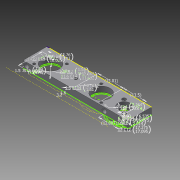
# Autodesk Inventor part: mount
Saved by Autodesk Inventor 2014 (Build 180170000, 170)
## iProperties
Created: 2013-09-13
Part Number: mount
Material: Generic
Document SubType Name: Modeling
Designer: Brandon
Density: 1 g/cm^3
Appearance: Default
Author: Brandon
Autodesk Inventor part; units mm, degrees
ref_plane "YZ Plane" through (0, 0, 0) normal (1, 0, 0) x (0, 1, 0)
ref_plane "XZ Plane" through (0, 0, 0) normal (0, 1, 0) x (-1, 0, 0)
ref_plane "XY Plane" through (0, 0, 0) normal (0, 0, 1) x (1, 0, 0)
sketch "Sketch1" plane through (0, 0, 0) normal (0, 0, 1) x (1, 0, 0)
  circle A0 centre (0, 0) radius 0.88
  circle A1 centre (-13, 0) radius 6.031
  line L0 (0, 7.8471) -> (0, -6.1529)
  line L1 (-22.031, -6.1529) -> (35.1375, -6.1529)
  line L2 (-22.031, 7.8471) -> (-22.031, -6.1529)
  circle A2 centre (-13, 0) radius 5.1925
  line L3 (-13, 0) -> (-9.1435, 0) construction
  line L4 (-13, 0) -> (-8.3268, 0) construction
  circle A3 centre (-8.1698, 4.8302) radius 0.775
  circle A4 centre (-17.8302, -4.8302) radius 0.75
  circle A5 centre (13, 0) radius 6.031
  circle A6 centre (13, 0) radius 5.1925
  line L5 (13, 0) -> (9.1435, 0) construction
  line L6 (13, 0) -> (8.3268, 0) construction
  circle A7 centre (8.1698, 4.8302) radius 0.775
  circle A8 centre (17.8302, -4.8302) radius 0.75
  line L7 (13, 0) -> (-13, 0)
  circle A9 centre (26.5, 0) radius 4.5 construction
  circle A10 centre (26.5, 0) radius 8.6375
  line L8 (26.5, 0) -> (30.5894, 0) construction
  circle A11 centre (22.8938, 3.6062) radius 1.132
  circle A12 centre (30.1062, -3.6062) radius 1.132
  line L9 (0, -6.1529) -> (-0.0044, -7.7529) construction
  line L10 (-0.0044, -7.7529) -> (-19.5609, -7.6995) construction
  line L11 (-0.0044, -7.7529) -> (19.5522, -7.8064) construction
  circle A13 centre (13, 0) radius 9 construction
  circle A14 centre (26.5, 0) radius 2.5 construction
  circle A15 centre (26.5, 0) radius 3.2675
  line L12 (13, 0) -> (26.5, 0)
  line L13 (30.1062, -3.6062) -> (22.8938, 3.6062) construction
  line L14 (33.2882, -0.4243) -> (26.0757, 6.7882)
  line L15 (19.7118, 0.4243) -> (26.9243, -6.7882)
  arc A16 (26.9243, -6.7882) -> (33.2882, -0.4243) centre (30.1062, -3.6062) ccw
  arc A17 (26.0757, 6.7882) -> (19.7118, 0.4243) centre (22.8938, 3.6062) ccw
  circle A18 centre (26.5, 0) radius 7.7
  circle A19 centre (26.5, 0) radius 3.5
  line L16 (-22.031, 7.8471) -> (35.1375, 7.8471)
  line L17 (35.1375, 7.8471) -> (35.1375, -6.1529)
  line L18 (20.438, -6.1529) -> (32.562, -6.1529) construction
  line L19 (-0.0044, -7.7529) -> (-0.0007, -10.9529) construction
  line L20 (-0.0007, -10.9529) -> (30.0115, -10.9189) construction
  line L21 (-0.0007, -10.9529) -> (-30.0007, -10.9869) construction
  line L22 (-0.0007, -10.9529) -> (29.9993, -10.9529) construction
  circle A20 centre (0, 0) radius 4 construction
  line L23 (-13, 0) -> (-8.7354, 4.2646) construction
  line L24 (-13, 0) -> (-17.2646, -4.2646) construction
  line L25 (-8.7354, 4.2646) -> (-8.1698, 4.8302) construction
  line L26 (-17.2646, -4.2646) -> (-17.8302, -4.8302) construction
  line L27 (-17.2646, -4.2646) -> (-16.4646, -4.2646) construction
  circle A21 centre (13, 0) radius 12 construction
  circle A22 centre (-13, 0) radius 12 construction
  line L28 (1, 0) -> (-1, 0) construction
  line L29 (-19.031, 0) -> (-22.031, 0) construction
  dimension "d105" = 24
  dimension "d106" = 24
  dimension "d0" = 1.5
  dimension "d3" = 11.6
  dimension "d8" = 10
  dimension "d13" = 1.5
  dimension "d14" = 1.5
  dimension "d26" = 17
  dimension "d31" = 2
  dimension "d32" = 2
  dimension "d38" = 5
  dimension "d40" = 6.15
  dimension "d42" = 13
  dimension "d52" = 13.5
  dimension "d53" = 9
  dimension "d54" = 7
  dimension "d60" = 12.124
  dimension "d81" = 1.6
  dimension "d86" = 3.2
  dimension "d87" = 45
  dimension "d88" = 10.2
  dimension "d89" = 8
  dimension "d90" = 0.8
  dimension "d91" = 0.8
  dimension "d92" = 135
  dimension "d98" = 14
  dimension "d103" = 18
  dimension "d104" = 9
  dimension "d107" = 2
  dimension "d108" = 3
  constraints: 62 end point, 21 centre point, 15 coincident, 9 point on circle, 8 horizontal, 7 collinear, 7 point on line, 7 tangent, 6 symmetric about line, 4 perpendicular, 2 equal length, 2 horizontal alignment, 2 midpoint, 1 parallel, 8 other
  measures "d14" diameter of A4
  measures "d38" diameter of A14
  measures "d42" distance of point (0, 0) A5.centre
  measures "d52" distance of L12.start L8.start
  measures "d53" diameter of A17
  measures "d54" diameter of A19
  measures "d60" distance of L18.start L18.end
  measures "d81" distance of L9.end L0.end
  measures "d86" distance of L9.end L19.end
  measures "d87" angle of L8 L13
  measures "d88" distance of L13.start L13.end
  measures "d89" diameter of A20
  measures "d90" distance of L23.end L25.end
  measures "d91" distance of L24.end L26.end
  measures "d92" angle of L26 L27
  measures "d98" distance of L2.start L1.start
  measures "d103" diameter of A13
  measures "d104" diameter of A9
  measures "d107" distance of L28.start L28.end
  measures "d108" distance of L29.start L29.end
extrude "Extrusion5" add sketch "Sketch1" along normal blind 4 contours L7 L0 A0 | L7 A5 A10 L1 L0 A0 | A0 L0 L16 A17 A10 A5 L7 | A0 L0 L7 | L0 L7 A0 | A0 L0 L1 L2 L16 | A0 L7 L0 | L7 A6 A10 A5 | A5 A10 A6 L7 | A10 A17 A5 | A5 A18 L12 A6 A10 | A10 A6 L12 A18 A5 | A5 A18 L1 A10 | L16 A10 A17 | A17 A18 A5 | A17 A10 L16 A18 | A18 L12 A5 | A5 L12 L15 L1 A18 | A18 A17 L15 L12 A5 | A5 L12 A18 | A18 A17 L14 A16 L1 L15 | L16 L17 A10 | A10 A16 A18 A17 L16 | A10 A16 L1 | L1 A18 A16 A10 | A16 A10 L17 L1 | A18 A16 L14 A17 | A1 picked at (20.7047, 6.7683) picked at (33.2521, -5.8435) picked at (32.0585, -5.7172)
extrude "Extrusion6" add sketch "Sketch1" along normal blind 0.6 contours A19
extrude "Extrusion7" add sketch "Sketch1" against normal blind 1 contours A18 L12 A5 | A5 L12 L15 L1 A18 | L1 L15 A16 A18 | A18 A17 L15 L12 A5 | A5 L12 A18 | A18 A17 L14 A16 L1 L15 | L1 A18 A16 L15 | A18 A16 L14 A17 | A19
extrude "Extrusion8" add sketch "Sketch1" against normal blind 2 contours L16 A10 A17 | A17 A10 L16 | A17 A10 L16 A18 | A17 L16 A10 | A16 A18 L1 A10 | A10 L1 A16 | A18 A17 L14 A16 L1 L15 | L1 A18 A16 L15 | A10 A16 L1 | L1 A18 A16 A10 | A19 picked at (20.7047, 6.7683) picked at (22.1116, 7.9072) picked at (23.7903, 7.8802) picked at (31.146, -6.8855) picked at (29.1888, -6.3623) picked at (32.0585, -5.7172)
extrude "Extrusion9" cut sketch "Sketch1" against normal up to surface (1 mm away) from surface at -1 contours A10 A17 A5 | A5 A18 L12 A6 A10 | A10 A6 L12 A18 A5 | A5 A18 L1 A10 | A17 A18 A5 | A17 A10 L16 A18 | A6 L12 A10 | A18 L12 A5 | A5 L12 L15 L1 A18 | A10 L12 A6 | A17 L16 A10 | A10 L16 A17 | A18 A17 L15 L12 A5 | A5 L12 A18 | A18 A17 L14 A16 L1 L15 | A10 A16 A18 A17 L16 | L1 A18 A16 A10 | A18 A16 L14 A17 | A19 picked at (23.7903, 7.8802) picked at (27.6663, 8.0331) picked at (32.0585, -5.7172)
extrude "Extrusion10" cut sketch "Sketch1" against normal blind 2 contours L7 L0 A0 | L7 A5 A10 L1 L0 A0 | A0 L0 L16 A17 A10 A5 L7 | A0 L0 L7 | A10 A17 A5 | A5 A18 L1 A10 | L16 A10 A17 | A17 A18 A5 | A17 A10 L16 A18 | A5 L12 L15 L1 A18 | A18 A17 L15 L12 A5 | A18 A17 L14 A16 L1 L15 | L16 L17 A10 | A10 A16 A18 A17 L16 | A10 A16 L1 | L1 A18 A16 A10 | A16 A10 L17 L1 | A18 A16 L14 A17 keep common part picked at (0.4122, 0.4122) picked at (0.4122, -0.4122) picked at (20.7047, 6.7683) picked at (33.2521, -5.8435) picked at (32.0585, -5.7172)
extrude "Extrusion11" add sketch "Sketch1" along normal blind 4 contours L7 L0 A0 | L7 A5 A10 L1 L0 A0 | A0 L0 L16 A17 A10 A5 L7 | A0 L0 L7 | L0 L7 A0 | A0 L0 L1 L2 L16 | A0 L7 L0 | L7 A6 A10 A5 | A5 A10 A6 L7 | A10 A17 A5 | A5 A18 L12 A6 A10 | A10 A6 L12 A18 A5 | A5 A18 L1 A10 | L16 A10 A17 | A17 A18 A5 | A17 A10 L16 A18 | A18 L12 A5 | A5 L12 L15 L1 A18 | A18 A17 L15 L12 A5 | A5 L12 A18 | A18 A17 L14 A16 L1 L15 | L16 L17 A10 | A10 A16 A18 A17 L16 | A10 A16 L1 | L1 A18 A16 A10 | A16 A10 L17 L1 | A18 A16 L14 A17 | A1 picked at (20.7047, 6.7683) picked at (33.2521, -5.8435) picked at (32.0585, -5.7172)
extrude "Extrusion12" add sketch "Sketch1" against normal blind 1 contours A19
extrude "Extrusion13" add sketch "Sketch1" along normal blind 0.5 contours A19
extrude "Extrusion14" cut sketch "Sketch1" along normal blind 0.9 contours L7 A6 A10 A5 | A5 A10 A6 L7 | A5 A18 L12 A6 A10 | A10 A6 L12 A18 A5 | A18 L12 A5 | A5 L12 A18 | A1
extrude "Extrusion15" cut sketch "Sketch1" along normal blind 10 contours L7 L0 A0 | A0 L0 L7 | L0 L7 A0 | A0 L7 L0
sketch "Sketch2" plane through (22.8903, 7.8471, -1) normal (0, 1, 0) x (1, 0, 0)
  line L0 (12.2472, -5) -> (-44.9213, -5) projected
  line L1 (-40.9213, -1) -> (-44.9213, -1)
  line L2 (-44.9213, -1) -> (-44.9213, -5)
  circle A0 centre (-43.9213, -3) radius 1.38
  line L3 (-22.8903, -1) -> (-22.8903, -5)
  circle A1 centre (-1.8593, -3) radius 1.38
  dimension "d95" = 4
  dimension "d97" = 2.5
  constraints: 6 end point, 2 centre point, 1 perpendicular, 1 point on line, 1 symmetric about line, 1 other
  measures "d95" distance of L1.end L1.start
extrude "Extrusion16" cut sketch "Sketch2" against normal blind 14 contours A0 L2 | L2 A0
extrude "Extrusion17" cut sketch "Sketch2" against normal blind 14 contours A1
body "Solid3"
